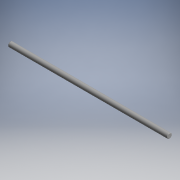
# Autodesk Inventor part: SSFMR10-330_s
Saved by Autodesk Inventor 2017.3 (Build 213256000, 256)
## iProperties
Part Number: SSFMR10-330_s
Material: Generic
Catalog Web Link: www.cadenas.de
Description: NSFMR, SFMR, PSFMR, SSFMR, NSFHR, SFHR, PSFHR, SSFHR, NSFR, SFR, PSFR, SSFR, HFR, PHFR_shaft-Rotary Shafts - Straight -
Vendor: MISUMI
Document SubType Name: Modeling
Designer: partserver
Manufacturer: MISUMI
Mass: 25.9105 g
Surface Area: 105.053 cm^2
Volume: 25.9105 cm^3
Density: 1 g/cm^3
Appearance: PSOLRGB-192-192-192
Category: PARTsolutions
Company: MISUMI
Title: SSFMR10-330
Author: Cadenas PARTsolutions
Comments: Rotary Shafts - Straight -
PSOL_IDENT_0: {$CADENAS_DATA\23d-libs\misumi\metric\11_rotary_shafts\11_components\psfr\psfr.prj},462 {VTYP=3D},{N
PSOL_IDENT_1: B=SSFMR10-330_s},{LINA=SSFMR10-330},{NN=NSFMR, SFMR, PSFMR, SSFMR, NSFHR, SFHR, PSFHR, SSFHR, NSFR,
PSOL_IDENT_2: SFR, PSFR, SSFR, HFR, PHFR_shaft},{DATE=02.06.2021 03:58:48},{GEOMDATE=05.02.2021 07:23:42},{VERSION=
PSOL_IDENT_3: },{LINEID=30},{WBVAR=TS,MAT,ST,ALT1,L,ALT2,KC,A,WKC,C,K,E,KZ,Z,ALT3,FC,GALT3,WFC,J,WALT3,V,ALT4,SFC,
PSOL_IDENT_4: SG,AG,ALT10,KWC,ALT11,WC,ALT6,TA,TB,ALT5,UC,ALT7,SC,ALT32,CD},{WBNUMERIC=L,KC,A,WKC,C,K,E,KZ,Z,FC,GA
PSOL_IDENT_5: LT3,WFC,J,WALT3,V,SFC,SG,AG,KWC,WC,TA,TB,UC,SC}  {NB=SSFMR10-330_s},{LINA=SSFMR10-330},{KT=DUMMY},{P
PSOL_IDENT_6: N=SSFMR10-330},{TYPE=SSFMR},{TS=M},{TSALG= 'M','h9 (Cold-drawn)','H','h7 (Ground)','','g6 (Ground)'
PSOL_IDENT_7: },{MAT=SUS304},{MATALG= 'S45C','S45C Equivalent', 'SUS304','SUS304' },{ST=-},{STALG= '-','-' },{D=10
PSOL_IDENT_8: .0},{ALT1=},{L=330.0},{LALG=[15:800/0.1]},{LMIN=15},{LMAX=800},{ALT2=},{ALT2ALG= '', 'w/o Key Groove
PSOL_IDENT_9: s','KC','with KC (Key Groove)','WKC','with WKC (Two Key Grooves)','KCWKC','with KC + WKC (Three Key
PSOL_IDENT_10: Grooves)','KZ','with KC + WKC + KZ (Four Key Grooves)' },{ALT2PN=},{KC=0.0},{KCALG=[0]},{KCMIN=0},{K
PSOL_IDENT_11: CMAX=0},{A=0.0},{AALG=[0]},{AMIN=3},{AMAX=0},{WKC=0.0},{WKCALG=[0]},{WKCMIN=0},{WKCMAX=0},{C=0.0},{C
PSOL_IDENT_12: ALG=[0]},{CMIN=3},{CMAX=0},{K=0.0},{KALG=[0]},{KMIN=0},{KMAX=325},{E=0.0},{EALG=[0]},{EMIN=3},{EMAX=
PSOL_IDENT_13: 100},{KZ=0.0},{KZALG=[0]},{KZMIN=332},{KZMAX=327},{Z=0.0},{ZALG=[0]},{ZMIN=3},{ZMAX=100},{CIFKC=1},{
PSOL_IDENT_14: CIFWKC=1},{CIFK=1},{CIFKZ=2},{PCUT3D=0.000},{QCUT3D=0},{BB=3},{BBALT2=3},{TT=1.8},{TTALT2=1.8},{ALT3=
PSOL_IDENT_15: },{ALT3ALG= '', 'w/o Set Screw Flat','FC','with FC (Adds a Set Screw Flat)','WFC','with WFC (Adds Tw
PSOL_IDENT_16: o Set Screw Flats)','FCWFC','with FC + WFC (Adds Three Set Screw Flats)' },{ALT3PN=},{FC=0},{FCALG=[
PSOL_IDENT_17: 0]},{FCMIN=0},{FCMAX=329},{GALT3=0},{GALT3ALG=[0]},{GALT3MIN=1},{GALT3MAX=70},{GALT3MAX2=70},{GALT3M
PSOL_IDENT_18: AX3=70},{WFC=0},{WFCALG=[0]},{WFCMIN=0},{WFCMIN2=2},{WFCMAX=326},{WFCMAX2=-3},{WFCMAX3=-4},{J=0},{JA
PSOL_IDENT_19: LG=[0]},{JMIN=1},{JMAX=70},{JMAX2=-2},{JMAX3=-5},{WALT3=0},{WALT3ALG=[0]},{WALT3MIN=0},{WALT3MIN2=33
PSOL_IDENT_20: 2},{WALT3MAX=327},{WALT3MAX2=327},{WALT3MAX3=327},{V=0},{VALG=[0]},{VMIN=1},{VMAX=70},{VMAX2=70},{VM
PSOL_IDENT_21: AX3=50},{CIFFC=0},{ALT4=},{ALT4ALG= '', 'w/o SFC (2 Set Screw Flats (Angle Specified))', 'SFC'  , 'w
PSOL_IDENT_22: ith SFC (2 Set Screw Flats (Angle Specified))'},{ALT4PN=},{SFC=0},{SFCALG=[0]},{SFCMIN=0},{SFCMAX=32
PSOL_IDENT_23: 9},{SG=0},{SGALG=[0]},{SGMIN=1},{SGMAX=70},{AG=0},{AGALG=[0]},{H=0.0},{CIFSFC=0},{ALT10=},{ALT10ALG=
PSOL_IDENT_24: '', 'w/o KWC (2 Set Screw Flats at both ends)', 'KWC', 'with KWC (2 Set Screw Flats at both ends)'
PSOL_IDENT_25: },{ALT10PN=},{KWC=0},{KWCALG=[0]},{KWCMIN=1},{KWCMAX=164},{WALT10=8},{ALT11=},{ALT11ALG= '','Not app
PSOL_IDENT_26: licable' },{ALT11PN=},{WC=0.0},{WCALG=[0]},{ALT6=},{ALT6ALG= '','w/o Retaining Ring Groove','TA','wi
PSOL_IDENT_27: th TA (Retaining Ring Groove)','TB','with TB (Retaining Ring Groove)','TATB','with TA + TB (Two Reta
PSOL_IDENT_28: ining Ring Grooves)' },{ALT6PN=},{TA=0.0},{TAALG=[0]},{TAMIN=2},{TAMAX=0},{TB=0.0},{TBALG=[0]},{TBMI
PSOL_IDENT_29: N=2},{TBMAX=0},{DDALT6=0.0},{MM=0.00},{ALT5=},{ALT5ALG= '', 'w/o UC (Slit Cam Groove)', 'UC', 'with
PSOL_IDENT_30: UC (Slit Cam Groove)'},{ALT5PN=},{UC=0},{UCALG=[0]},{UCMIN=1},{UCMAX=324},{DDALT5=0},{LL1=0},{ALT7=}
PSOL_IDENT_31: ,{ALT7ALG= '', 'w/o SC (Wrench Flats)', 'SC', 'with SC (Wrench Flats)'},{ALT7PN=},{SC=0},{SCALG=[0]}
PSOL_IDENT_32: ,{SCMIN=0},{SCMAX=322},{WALT7=0},{LL2=0},{LL2ALG=8},{CIFSC=0},{ALT32=},{ALT32ALG=  '','w/o CD (Chang
PSOL_IDENT_33: es Part D Chamfering)','-CD', 'with CD (Changes Part D Chamfering)' },{ALT32PN=},{CD=},{CDALG= '','N
PSOL_IDENT_34: /A' },{CD3D=0.5},{CIF32=0},{CIF320=0},{CIFTA=0},{CIFTB=0},{ERRORPN=},{ERRORALT23=OK},{ERRORALT24=OK}
PSOL_IDENT_35: ,{ERRORALT25=OK},{ERRORALT26=OK},{ERRORALT27=OK},{ERRORALT210=OK},{ERRORALT34=OK},{ERRORALT35=OK},{E
PSOL_IDENT_36: RRORALT36=OK},{ERRORALT37=OK},{ERRORALT310=OK},{ERRORALT45=OK},{ERRORALT46=OK},{ERRORALT47=OK},{ERRO
PSOL_IDENT_37: RALT410=OK},{ERRORALT56=OK},{ERRORALT57=OK},{ERRORALT510=OK},{ERRORALT610=OK},{ERRORALT75=OK},{ERROR
PSOL_IDENT_38: ALT76=OK},{ERRORALT710=OK}
NB: SSFMR10-330_s
NN: NSFMR, SFMR, PSFMR, SSFMR, NSFHR, SFHR, PSFHR, SSFHR, NSFR, SFR, PSFR, SSFR, HFR, PHFR_shaft
NT: Rotary Shafts - Straight -
NBSYN: $PN._s
LINA: SSFMR10-330
CATALOG: Misumi
PN: SSFMR10-330
TS: h9 (Cold-drawn)
MAT: SUS304
ST: -
D: 10
ALT1: w/o LKC (Changes L Tolerance)
L: 330
ALT2: w/o Key Grooves
KC: 0
A: 0
WKC: 0
C: 0
K: 0
E: 0
KZ: 0
Z: 0
ALT3: w/o Set Screw Flat
FC: 0
GALT3: 0
WFC: 0
J: 0
WALT3: 0
V: 0
ALT4: w/o SFC (2 Set Screw Flats (Angle Specified))
SFC: 0
SG: 0
AG: 0
H: 0
ALT10: w/o KWC (2 Set Screw Flats at both ends)
KWC: 0
ALT11: Not applicable
WC: 0
ALT6: w/o Retaining Ring Groove
TA: 0
TB: 0
DDALT6: 0
MM: 0
ALT5: w/o UC (Slit Cam Groove)
UC: 0
DDALT5: 0
LL1: 0
ALT7: w/o SC (Wrench Flats)
SC: 0
WALT7: 0
LL2: 0
ALT32: w/o CD (Changes Part D Chamfering)
CD: N/A
SUPPLIER: MISUMI
ARTICLENO: SSFMR10-330_s
BOMINFO: SSFMR10-330
CREATOR: CADENAS GmbH
Autodesk Inventor part; units mm, degrees
ref_plane "YZ Plane" through (0, 0, 0) normal (1, 0, 0) x (0, 1, 0)
ref_plane "XZ Plane" through (0, 0, 0) normal (0, 1, 0) x (-1, 0, 0)
ref_plane "XY Plane" through (0, 0, 0) normal (0, 0, 1) x (1, 0, 0)
sketch "Sketch_1" plane through (0, 0, 0) normal (0, 0, 1) x (1, 0, 0)
  line L0 (330, 0) -> (0, 0)
  line L1 (0, 0) -> (0, 4.5)
  line L2 (0, 4.5) -> (0.5, 5)
  line L3 (0.5, 5) -> (329.5, 5)
  line L4 (329.5, 5) -> (330, 4.5)
  line L5 (330, 4.5) -> (330, 0)
  line L6 (330, 0) -> (0, 0)
  constraints: 14 end point
revolve "Revolution1" add sketch "Sketch_1" angle 360 about axis through (330, 0, 0) along (1, 0, 0)
ref_plane "COMBINATION_MODULE_XY" through (0, 0, 0) normal (1, 0, 0) x (0, 0, -1)
ref_plane "COMBINATION_MODULE_YZ" through (0, 0, 0) normal (0, 0, -1) x (0, 1, 0)
ref_plane "COMBINATION_MODULE_ZX" through (0, 0, 0) normal (0, 1, 0) x (1, 0, 0)
body "Solid1"
